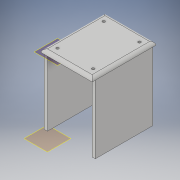
# Autodesk Inventor part: Relé - columnes tapa
Saved by Autodesk Inventor 2019 (Build 230136000, 136)
## iProperties
Created: 2018-08-23
Part Number: Relé - columnes tapa
Material: Genérico
Document SubType Name: Modeling
Designer: Albert Garangou Culebras
Density: 1 g/cm^3
Appearance: Valor por defecto
Author: Albert Garangou Culebras
Autodesk Inventor part; units mm, degrees
ref_plane "YZ Plane" through (0, 0, 0) normal (1, 0, 0) x (0, 1, 0)
ref_plane "XZ Plane" through (0, 0, 0) normal (0, 1, 0) x (-1, 0, 0)
ref_plane "XY Plane" through (0, 0, 0) normal (0, 0, 1) x (1, 0, 0)
ref_plane "Plano de trabajo1" through (0, 3, 0) normal (0, 1, 0) x (1, 0, 0)
ref_plane "Plano de trabajo2" through (4.2498, 73, -5.25) normal (0, 1, 0) x (1, 0, 0)
sketch "Boceto3" plane through (4.2498, 73, -5.25) normal (0, 1, 0) x (1, 0, 0)
  line L0 (37.7502, 51.75) -> (40.7502, 51.75)
  line L1 (-7.2498, -8.25) -> (40.7502, -8.25)
  line L2 (40.7502, -8.25) -> (40.7502, 51.75)
  line L3 (40.7502, 51.75) -> (-7.2498, 51.75)
  line L4 (-7.2498, 51.75) -> (-7.2498, -8.25)
  circle A0 centre (33.5, 43.5) radius 1.25
  circle A1 centre (33.5, 0) radius 1.25
  circle A2 centre (0, 43.5) radius 1.25
  circle A3 centre (0, 0) radius 1.25
  point P0 (-4.2498, -5.25)
  point P1 (37.7502, -5.25)
  point P2 (37.7502, 48.75)
  dimension "d39" = 2.5
  dimension "d40" = 2.5
  dimension "d41" = 2.5
  dimension "d42" = 2.5
  constraints: 10 end point, 4 centre point, 3 coincident, 2 parallel, 1 horizontal, 1 perpendicular
  measures "d39" diameter of A0
  measures "d40" diameter of A1
  measures "d41" diameter of A2
  measures "d42" diameter of A3
ref_plane "Plano de trabajo3" through (4.2498, 73, -5.25) normal (0, -1, 0) x (1, 0, 0)
sketch "Boceto5" plane through (4.2498, 73, -5.25) normal (0, -1, 0) x (1, 0, 0)
  line L0 (-4.2498, 5.25) -> (-4.2498, -48.75) projected
  line L1 (-4.2498, 5.25) -> (-4.2498, -48.75)
  line L2 (37.7502, -48.75) -> (37.7502, 5.25)
  line L3 (37.7502, 5.25) -> (37.7502, 8.25)
  line L4 (37.7502, -48.75) -> (37.7502, -51.75)
  line L5 (-4.2498, 5.25) -> (-7.2498, 5.25)
  line L6 (-4.2498, -48.75) -> (-7.2498, -48.75)
  line L7 (37.7502, -48.75) -> (40.7502, -48.75)
  line L8 (37.7502, 5.25) -> (40.7502, 5.25)
  line L9 (40.7502, 5.25) -> (40.7502, -48.75)
  line L10 (40.7502, -51.75) -> (40.7502, 8.25) projected
  line L11 (-7.2498, -48.75) -> (-7.2498, 5.25)
  line L12 (-7.2498, 8.25) -> (-7.2498, -51.75) projected
  constraints: 20 end point, 2 collinear, 1 horizontal, 1 parallel
extrude "Extrusión5" add sketch "Boceto5" along normal blind 64
extrude "Extrusión6" add sketch "Boceto3" along normal blind 3
fillet "Empalme3" radius 3 4 edges at (21, 76, 3) (-3, 76, -27) (45, 76, -27) (21, 76, -57)
